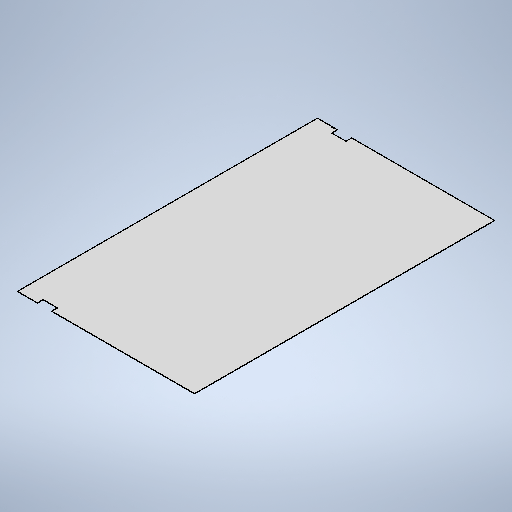
# Autodesk Inventor part: GnG frame 1.1 floor sheet 3
Saved by Autodesk Inventor 2025.3 (Build 293356000, 356)
## iProperties
Created: 2025-10-28
Part Number: GnG frame 1.1 floor sheet 3
Material: Stainless Steel
Document SubType Name: Sheet Metal
Designer: admin
Mass: 280.619 g
Surface Area: 364.406 cm^2
Volume: 35.0774 cm^3
Density: 8 g/cm^3
Sheet Metal Rule: AISI304 3mm Die 32
Sheet Metal Width: 1240,000 mm
Sheet Metal Length: 2100,000 mm
Sheet Metal Area: 2604000,000 mm^2
Appearance: Default
Stock Number: 1.3
Flat Pattern Width: 124 cm
Flat Pattern Length: 210 cm
Flat Pattern Area: 26040 cm^2
Author: admin
Autodesk Inventor part; units mm, degrees
ref_plane "YZ Plane" through (0, 0, 0) normal (1, 0, 0) x (0, 1, 0)
ref_plane "XZ Plane" through (0, 0, 0) normal (0, 1, 0) x (-1, 0, 0)
ref_plane "XY Plane" through (0, 0, 0) normal (0, 0, 1) x (1, 0, 0)
sketch "Sketch1" plane through (0, 0, 0) normal (0, 0, 1) x (1, 0, 0)
  line L0 (0, 0) -> (-1240, 0)
  line L1 (-1240, 0) -> (-1240, -2100)
  line L2 (-1240, -2100) -> (0, -2100)
  line L3 (0, -2100) -> (0, 0)
  line L4 (0, 0) -> (-40, 0)
  line L5 (-40, 0) -> (-40, -40)
  line L6 (-40, -40) -> (0, -40)
  line L7 (0, -40) -> (0, 0)
  line L8 (0, -2100) -> (-40, -2100)
  line L9 (-40, -2100) -> (-40, -2060)
  line L10 (-40, -2060) -> (0, -2060)
  line L11 (0, -2060) -> (0, -2100)
  line L12 (-1240, 0) -> (-1200, 0)
  line L13 (-1200, 0) -> (-1200, -40)
  line L14 (-1200, -40) -> (-1240, -40)
  line L15 (-1240, -40) -> (-1240, 0)
  line L16 (-1240, -2100) -> (-1200, -2100)
  line L17 (-1200, -2100) -> (-1200, -2060)
  line L18 (-1200, -2060) -> (-1240, -2060)
  line L19 (-1240, -2060) -> (-1240, -2100)
  line L20 (-1100, -2100) -> (-1000, -2100)
  line L21 (-1000, -2100) -> (-1000, -2060)
  line L22 (-1000, -2060) -> (-1100, -2060)
  line L23 (-1100, -2060) -> (-1100, -2100)
  line L24 (-1100, 0) -> (-1000, 0)
  line L25 (-1000, 0) -> (-1000, -40)
  line L26 (-1000, -40) -> (-1100, -40)
  line L27 (-1100, -40) -> (-1100, 0)
  point P0 (0, -40)
  point P1 (-40, 0)
  point P2 (-40, -2100)
  point P3 (0, -2060)
  point P4 (-1000, -2100)
  point P5 (-1000, 0)
  dimension "d22" = 1240
  dimension "d23" = 2100
  dimension "d24" = 40
  dimension "d25" = 40
  dimension "d28" = 100
  dimension "d29" = 960
  measures "d22" distance of L2.end L1.end
  measures "d23" distance of L1.end L0.end
  measures "d24" distance of L6.end L5.end
  measures "d25" distance of L5.end L4.end
  measures "d28" distance of L25.end L26.end
  measures "d29" distance between parallel lines of L5 L25
extrude "Plate1" add sketch "Sketch1" along normal blind 3 contours L3 L6 L5 L0 | L5 L6 L3 L10 L9 L2 L21 L22 L23 L17 L18 L1 L14 L13 L0 L27 L26 L25 | L3 L2 L9 L10 | L13 L14 L1 L0 | L18 L17 L2 L1
sketch "Sketch6" plane through (0, 0, 3) normal (0, 0, 1) x (1, 0, 0)
  line L0 (-1135, 0) -> (-1133, 0)
  line L1 (-1127, -5) -> (-1127, 0)
  line L2 (-1127, 0) -> (-1125, 0)
  line L3 (-1125, 0) -> (-1125, -5)
  line L4 (-1125, 0) -> (-1123, 0) construction
  line L5 (-1123, 0) -> (-1121.9884, -4.6072)
  arc A0 (-1121.9884, -4.6072) -> (-1121.0116, -4.6072) centre (-1121.5, -4.5) ccw
  line L6 (-1123, 0) -> (-1120, 0)
  line L7 (-1120, 0) -> (-1118, 0) construction
  line L8 (-1118, -5) -> (-1118, 0)
  line L9 (-1116, -5) -> (-1118, -5)
  line L10 (-1116, 0) -> (-1116, -5)
  line L11 (-1118, 0) -> (-1116, 0)
  line L12 (-1116, -2.5) -> (-1114, -2.5) construction
  line L13 (-1121.0116, -4.6072) -> (-1120, 0)
  line L14 (-1133, 0) -> (-1133, -5)
  line L15 (-1133, -5) -> (-1135, -5)
  line L16 (-1135, -5) -> (-1135, 0)
  line L17 (-1125, -5) -> (-1127, -5)
  line L18 (-1129, 0) -> (-1129, -5)
  line L19 (-1129, -5) -> (-1131, -5)
  line L20 (-1131, -5) -> (-1131, 0)
  line L21 (-1131, 0) -> (-1129, 0)
  line L22 (-1129, -2.5) -> (-1127, -2.5) construction
  line L23 (-1133, -2.5) -> (-1131, -2.5) construction
  line L24 (-1114, -5) -> (-1114, 0)
  line L25 (-1112, 0) -> (-1112, -5)
  line L26 (-1112, -5) -> (-1114, -5)
  line L27 (-1114, 0) -> (-1112, 0)
  line L28 (-1112, -2.5) -> (-1110, -2.5) construction
  line L29 (-1110, -5) -> (-1110, 0)
  line L30 (-1110, 0) -> (-1108, 0)
  line L31 (-1108, -5) -> (-1110, -5)
  arc A1 (-1141.5, 0) -> (-1138.5, 0) centre (-1140, 0) ccw
  line L32 (-1108, 0) -> (-1108, -5)
  line L33 (-1240, 0) -> (-1100, 0) projected
  line L34 (-1240, -2100) -> (-1240, 0) projected
  point P0 (0, 0)
  point P1 (-1121.5, 0)
  dimension "d38" = 2
  dimension "d39" = 5
  dimension "d40" = 0.5
  dimension "d41" = 3
  dimension "d42" = 2
  dimension "d43" = 5
  dimension "d44" = 3
  dimension "d45" = 5
  dimension "d46" = 100
  constraints: 66 end point, 12 parallel, 11 horizontal, 10 equal length, 9 midpoint, 6 perpendicular, 5 collinear, 4 point on circle, 4 point on line, 3 tangent, 2 centre point, 1 vertical alignment
  measures "d38" distance of L14.end L16.start
  measures "d39" distance of L16.start L0.start
  measures "d40" radius of A0
  measures "d41" distance of L5.start L6.end
  measures "d42" distance of L10.end L8.start
  measures "d43" distance of L8.start L7.end
  measures "d44" diameter of A1
  measures "d45" distance of A1.centre L0.start
  measures "d46" distance from line of L34 A1.centre
extrude "Cut1" cut sketch "Sketch6" against normal blind 3 contours L2 L3 L17 L1 | L21 L18 L19 L20 | L0 L14 L15 L16 | A1 L33
equation "\"d24\" = d25"
equation "\"d40\" = 0.25 * d38"
equation "\"d47\" = Thickness"
equation "\"d2\" = Thickness"
equation "\"BendReliefWidth\" = Thickness"
equation "\"BendReliefDepth\" = 0.5 * Thickness"
equation "\"CornerReliefSize\" = 4 * Thickness"
equation "\"MinimumRemnant\" = 2 * Thickness"
equation "\"TransitionRadius\" = BendRadius"
equation "\"JacobiRadiusSize\" = BendRadius"
equation "\"GapSize\" = Thickness"
equation "\"Thickness\" = 3"
equation "\"BendRadius\" = 5"
body "Solid1"
